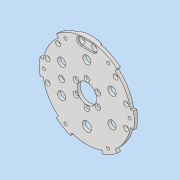
# Autodesk Inventor part: SpoolSectionSealingWallFront
Saved by Autodesk Inventor 2017 (Build 210142000, 142)
## iProperties
Created: 2016-11-06
Part Number: SpoolSectionSealingWallFront
Material: ABS Plastic
Document SubType Name: Modeling
Designer: techn
Density: 1.06 g/cm^3
Appearance: Smooth - White
Mass: 19.8709 g
Surface Area: 141.421 cm^2
Volume: 18.7461 cm^3
Author: techn
Autodesk Inventor part; units mm, degrees
ref_plane "YZ Plane" through (0, 0, 0) normal (1, 0, 0) x (0, 1, 0)
ref_plane "XZ Plane" through (0, 0, 0) normal (0, 1, 0) x (-1, 0, 0)
ref_plane "XY Plane" through (0, 0, 0) normal (0, 0, 1) x (1, 0, 0)
sketch "Sketch1" plane through (0, 0, 0) normal (0, 0, 1) x (1, 0, 0)
  circle A0 centre (0, 0) radius 47.625
  dimension "d0" = 95.25
  constraints: 1 centre point, 1 coincident
  measures "d0" diameter of A0
extrude "Extrusion1" add sketch "Sketch1" along normal blind 3.175
sketch "Sketch7" plane through (0, 0, 0) normal (0, 0, -1) x (-1, 0, 0)
  line L0 (0, 0) -> (0, 12.7)
  circle A0 centre (0, 12.7) radius 1.5875
  circle A1 centre (0, 12.7) radius 3.81
  circle A2 centre (-10.998523, 6.35) radius 3.81
  circle A3 centre (-10.998523, 6.35) radius 1.5875
  circle A4 centre (-10.998523, -6.35) radius 3.81
  circle A5 centre (-10.998523, -6.35) radius 1.5875
  circle A6 centre (0, -12.7) radius 3.81
  circle A7 centre (0, -12.7) radius 1.5875
  circle A8 centre (10.998523, -6.35) radius 3.81
  circle A9 centre (10.998523, -6.35) radius 1.5875
  circle A10 centre (10.998523, 6.35) radius 3.81
  circle A11 centre (10.998523, 6.35) radius 1.5875
  circle A12 centre (0, 0) radius 47.625
  dimension "d38" = 12.7
  dimension "d39" = 3.175
  dimension "d40" = 7.62
  dimension "d43" = 360
  dimension "d51" = 0
  constraints: 12 centre point, 8 coincident, 2 end point, 1 vertical, 25 other
  measures "d38" distance of L0.start L0.end
  measures "d39" diameter of A0
  measures "d40" diameter of A1
  measures "d51" distance of L0.start A12.centre
extrude "Extrusion8" cut sketch "Sketch7" against normal blind 6.35 contours A0 | A3 | A5 | A7 | A9 | A11
chamfer "Chamfer1" distance 1.27 angle 45 6 edges at (1.5875, 12.7, 3.175) (12.586, 6.35, 3.175) (12.586, -6.35, 3.175) (-9.411, 6.35, 3.175) (-9.411, -6.35, 3.175) (1.5875, -12.7, 3.175)
sketch "Sketch8" plane through (0, 0, 3.175) normal (0, 0, 1) x (1, 0, 0)
  line L0 (0, 0) -> (21.43125, 37.120014)
  line L1 (0, 0) -> (42.8625, 0) construction
  circle A0 centre (21.43125, 37.120014) radius 1.5875
  circle A1 centre (-21.43125, 37.120014) radius 1.5875
  circle A2 centre (-42.8625, 0) radius 1.5875
  circle A3 centre (-21.43125, -37.120014) radius 1.5875
  circle A4 centre (21.43125, -37.120014) radius 1.5875
  circle A5 centre (42.8625, 0) radius 1.5875
  dimension "d52" = 42.8625
  dimension "d53" = 60
  dimension "d54" = 3.175
  dimension "d57" = 360
  constraints: 6 centre point, 4 end point, 1 coincident, 1 equal length, 1 horizontal, 13 other
  measures "d52" distance of L0.start L0.end
  measures "d53" angle of L1 L0
  measures "d54" diameter of A0
extrude "Extrusion9" cut sketch "Sketch8" against normal blind 25.4
sketch "Sketch9" plane through (0, 0, 3.175) normal (0, 0, 1) x (1, 0, 0)
  circle A0 centre (0, -28.575) radius 4.7625
  point P0 (0, 0)
  dimension "d61" = 9.525
  dimension "d62" = 28.575
  constraints: 1 centre point
  measures "d61" diameter of A0
  measures "d62" distance of A0.centre point (0, 0)
extrude "Extrusion10" cut sketch "Sketch9" against normal blind 25.4
sketch "Sketch11" plane through (0, 0, 3.175) normal (0, 0, 1) x (1, 0, 0)
  line L0 (0, 0) -> (16.288709, 44.752861)
  line L1 (0, 0) -> (47.625, 0) construction
  line L2 (0, 0) -> (-16.288709, 44.752861)
  arc A0 (16.288709, 44.752861) -> (-16.288709, 44.752861) centre (0, 0) ccw
  arc A1 (15.202795, 41.769337) -> (-15.202795, 41.769337) centre (0, 0) ccw
  dimension "d67" = 47.625
  dimension "d68" = 70
  dimension "d69" = 47.625
  dimension "d70" = 110
  dimension "d71" = 3.175
  dimension "d72" = 3.175
  dimension "d73" = 47.625
  dimension "d74" = 44.45
  constraints: 6 end point, 4 point on circle, 2 centre point, 2 point on line, 1 equal length, 1 horizontal
  measures "d67" distance of L0.start L0.end
  measures "d68" angle of L1 L0
  measures "d69" distance of L0.start L2.end
  measures "d70" angle of L1 L2
  measures "d71" distance of L2.end A1.end
  measures "d72" distance of L0.end A1.start
  measures "d73" radius of A0
  measures "d74" radius of A1
extrude "Extrusion11" cut sketch "Sketch11" against normal blind 25.4 contours A1 L2 A0 L0
pattern_circular "Circular Pattern1" count 6 over 360 about axis through (0, 0, 0) along (0, 0, 1) of "Extrusion11"
sketch "Sketch12" plane through (0, 0, 3.175) normal (0, 0, 1) x (1, 0, 0)
  line L0 (0, 0) -> (-25.4, 0)
  circle A0 centre (-25.4, 0) radius 3
  dimension "d80" = 25.4
  dimension "d81" = 6
  constraints: 2 end point, 1 centre point, 1 coincident, 1 horizontal
  measures "d80" distance of L0.start L0.end
  measures "d81" diameter of A0
extrude "Extrusion12" cut sketch "Sketch12" against normal blind 3.175
sketch "Sketch13" plane through (0, 0, 0) normal (0, 0, -1) x (-1, 0, 0)
  circle A0 centre (25.4, 0) radius 3 projected
  circle A1 centre (25.4, 0) radius 7.9375
  point P0 (0, 0)
  dimension "d84" = 15.875
  constraints: 1 centre point, 1 coincident
  measures "d84" diameter of A1
extrude "Extrusion13" add sketch "Sketch13" along normal blind 3.175 contours A0 | A1
fillet "Fillet1" radius 3.175 2 edges at (-17.4625, 0, 0) (-17.4625, 0, -3.175)
sketch "Sketch14" plane through (0, 0, 3.175) normal (0, 0, 1) x (1, 0, 0)
  line L0 (0, 0) -> (0, 29.21)
  circle A0 centre (0, 29.21) radius 4.1275
  circle A1 centre (-25.296602, 14.605) radius 4.1275
  circle A2 centre (-25.296602, -14.605) radius 4.1275
  circle A3 centre (0, -29.21) radius 4.1275
  circle A4 centre (25.296602, -14.605) radius 4.1275
  circle A5 centre (25.296602, 14.605) radius 4.1275
  circle A6 centre (0, 0) radius 9.8425
  circle A7 centre (-10.998523, 6.35) radius 2.8575
  dimension "d88" = 29.21
  dimension "d89" = 8.255
  dimension "d92" = 360
  constraints: 7 centre point, 2 coincident, 2 end point, 1 tangent, 1 vertical, 13 other
  measures "d88" distance of L0.start L0.end
  measures "d89" diameter of A0
extrude "Extrusion14" cut sketch "Sketch14" against normal through all contours A0 | A1 | A2 | A4 | A5 | A6
sketch "Sketch15" plane through (0, 0, 3.175) normal (0, 0, 1) x (1, 0, 0)
  arc A0 (-16.288709, 44.752861) -> (-30.61276, 36.482867) centre (0, 0) ccw
  arc A1 (15.202795, 41.769337) -> (-15.202795, 41.769337) centre (0, 0) ccw
  arc A2 (30.61276, 36.482867) -> (16.288709, 44.752861) centre (0, 0) ccw
  arc A3 (16.288709, 44.752861) -> (-16.288709, 44.752861) centre (0, 0) ccw
  line L0 (-15.202795, 41.769337) -> (-16.288709, 44.752861)
  line L1 (15.202795, 41.769337) -> (16.288709, 44.752861)
  constraints: 4 end point, 2 point on circle, 1 centre point, 1 concentric
extrude "Extrusion15" add sketch "Sketch15" against normal up to surface (3.175 mm away)
sketch "Sketch16" plane through (0, 0, 3.175) normal (0, 0, 1) x (1, 0, 0)
  line L0 (0, 0) -> (6.35, 42.32531)
  line L1 (0, 0) -> (-6.35, 42.32531)
  line L2 (-6.35, 42.32531) -> (6.35, 42.32531)
  circle A0 centre (6.35, 42.32531) radius 3.175
  circle A1 centre (-6.35, 42.32531) radius 3.175
  dimension "d98" = 42.799
  dimension "d99" = 42.799
  dimension "d100" = 12.7
  dimension "d101" = 6.35
  dimension "d102" = 6.35
  constraints: 6 end point, 2 centre point, 2 coincident, 1 horizontal
  measures "d98" distance of L0.start L0.end
  measures "d99" distance of L0.start L1.end
  measures "d100" distance of L1.end L0.end
  measures "d101" diameter of A0
  measures "d102" diameter of A1
extrude "Extrusion16" cut sketch "Sketch16" against normal blind 25.4 contours A0 L2 L0 | L0 L2 A0 | A1 L2 L1 | L1 L2 A1
sketch "Sketch17" plane through (0, 0, 0) normal (0, 0, -1) x (-1, 0, 0)
  circle A0 centre (-6.35, 42.32531) radius 3.175
  circle A1 centre (6.35, 42.32531) radius 3.175
  arc A2 (30.61276, 36.482867) -> (-30.61276, 36.482867) centre (0, 0) ccw
  circle A3 centre (-6.35, 42.32531) radius 4.826
  circle A4 centre (6.35, 42.32531) radius 4.826
  line L0 (-6.35, 37.49931) -> (6.35, 37.49931)
  arc A5 (7.066024, 47.097897) -> (-7.066024, 47.097897) centre (0, 0) ccw
  dimension "d105" = 9.652
  dimension "d106" = 9.652
  constraints: 8 point on circle, 3 centre point, 2 coincident, 2 end point, 1 concentric, 1 tangent
  measures "d105" diameter of A3
  measures "d106" diameter of A4
extrude "Extrusion17" add sketch "Sketch17" along normal blind 1.5875
chamfer "Chamfer2" distance 1.5875 angle 45 3 edges at (11.1626, 41.9663, 0) (0, 37.4993, 0) (-11.1626, 41.9663, 0)
sketch "Sketch18" plane through (0, 0, 3.175) normal (0, 0, 1) x (1, 0, 0)
  circle A0 centre (-6.35, 42.32531) radius 3.175
  circle A1 centre (6.35, 42.32531) radius 3.175
  circle A2 centre (-6.35, 42.32531) radius 4.1275
  circle A3 centre (6.35, 42.32531) radius 4.1275
  line L0 (-6.35, 38.19781) -> (6.35, 38.19781)
  line L1 (-6.35, 46.45281) -> (6.35, 46.45281)
  point P0 (0, 0)
  dimension "d112" = 8.255
  dimension "d113" = 8.255
  constraints: 4 end point, 4 point on circle, 2 centre point, 2 coincident, 2 horizontal, 1 tangent
  measures "d112" diameter of A2
  measures "d113" diameter of A3
extrude "Extrusion18" cut sketch "Sketch18" against normal blind 1.5875
sketch "Sketch19" plane through (0, 0, 3.175) normal (0, 0, 1) x (1, 0, 0)
  line L0 (0, 0) -> (39.377898, 10.551276)
  line L1 (0, 0) -> (40.767, 0) construction
  circle A0 centre (39.377898, 10.551276) radius 2.54
  line L2 (0, 0) -> (0, 7.899337)
  circle A1 centre (39.377898, -10.551276) radius 2.54
  circle A2 centre (-39.377898, 10.551276) radius 2.54
  circle A3 centre (-39.377898, -10.551276) radius 2.54
  line L3 (0, 0) -> (28.826622, 28.826622)
  line L4 (0, 0) -> (40.767, 0) construction
  circle A4 centre (28.826622, 28.826622) radius 2.54
  circle A5 centre (-28.826622, 28.826622) radius 2.54
  dimension "d116" = 40.767
  dimension "d117" = 15
  dimension "d118" = 5.08
  dimension "d121" = 40.767
  dimension "d122" = 45
  dimension "d123" = 5.08
  constraints: 10 end point, 6 centre point, 4 symmetric about line, 2 coincident, 2 equal length, 2 horizontal, 1 vertical, 4 other
  measures "d116" distance of L0.start L0.end
  measures "d117" angle of L1 L0
  measures "d118" diameter of A0
  measures "d121" distance of L0.start L3.end
  measures "d122" angle of L4 L3
  measures "d123" diameter of A4
extrude "Extrusion19" cut sketch "Sketch19" against normal blind 25.4 contours A0 | A1 | A2 | A3
extrude "Extrusion20" cut sketch "Sketch19" against normal blind 25.4 contours A4 | A5
equation "\"d99\" = d98"
body "Solid1"
